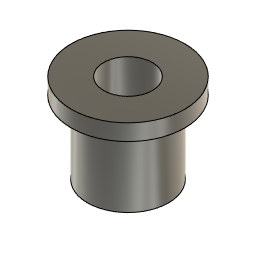
M3 v1 (Autodesk Fusion 360 design; units mm, degrees)
Autodesk Fusion 360 part; units mm, degrees
sketch "Esquisse1" plane through (0, 0, 0) normal (0, 0, 1) x (1, 0, 0)
  circle A0 centre (0, 0) radius 1.5
  circle A1 centre (0, 0) radius 2.5
  dimension "d1" = 3
  dimension "d2" = 5
  constraint coincident A0.centre A1.centre
  measures "d1" diameter of A0
  measures "d2" diameter of A1
extrude "Extrusion1" add sketch "Esquisse1" along normal blind 4.5
sketch "Esquisse2" plane through (0, 0, 4.5) normal (0, 0, 1) x (-1, 0, 0)
  circle A0 centre (0, 0) radius 1.5
  circle A1 centre (0, 0) radius 2.5
  circle A2 centre (0, 0) radius 1.5
  circle A3 centre (0, 0) radius 2.5
  circle A4 centre (0, 0) radius 3.5
  dimension "d5" = 3
  dimension "d6" = 5
  dimension "d7" = 7
  constraint concentric A0 A2
  constraint concentric A0 A3
  constraint concentric A2 A4
  measures "d5" diameter of A2
  measures "d6" diameter of A3
  measures "d7" diameter of A4
extrude "Extrusion2" add sketch "Esquisse2" along normal blind 1 contours A1 A3 | A4
